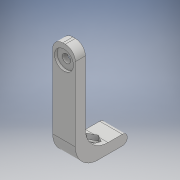
# Autodesk Inventor part: U2
Saved by Autodesk Inventor 2019 (Build 230136000, 136)
## iProperties
Part Number: U2
Material: Genérico
Document SubType Name: Modeling
Designer: beta3
Density: 1 g/cm^3
Appearance: Valor por defecto
Author: beta3
Autodesk Inventor part; units mm, degrees
ref_plane "YZ Plane" through (0, 0, 0) normal (1, 0, 0) x (0, 1, 0)
ref_plane "XZ Plane" through (0, 0, 0) normal (0, 1, 0) x (-1, 0, 0)
ref_plane "XY Plane" through (0, 0, 0) normal (0, 0, 1) x (1, 0, 0)
sketch "Boceto1" plane through (0, 0, 0) normal (0, 0, 1) x (1, 0, 0)
  line L0 (-13.5, 62) -> (13.5, 62)
  line L1 (13.5, 62) -> (13.5, 0)
  line L2 (13.5, 0) -> (-13.5, 0)
  line L3 (-13.5, 0) -> (-13.5, 62)
  line L4 (0, 0) -> (0, 62) construction
  line L5 (0, 40.815) -> (8.5, 35.9075)
  line L6 (8.5, 35.9075) -> (8.5, 26.0925)
  line L7 (8.5, 26.0925) -> (0, 21.185)
  line L8 (0, 21.185) -> (-8.5, 26.0925)
  line L9 (-8.5, 26.0925) -> (-8.5, 35.9075)
  line L10 (-8.5, 35.9075) -> (0, 40.815)
  line L11 (-8.5, 35.9075) -> (-13.5, 35.9075) construction
  line L12 (8.5, 35.9075) -> (13.5, 35.9075) construction
  point P0 (0, 31)
  dimension "d20" = 17
  dimension "d21" = 5
  dimension "d22" = 27
  dimension "d23" = 62
  constraints: 26 end point, 4 point on line, 3 midpoint, 2 parallel, 2 perpendicular, 1 horizontal, 1 symmetric about line, 1 vertical, 13 other
  measures "d20" distance between parallel lines of L6 L9
  measures "d21" distance of L9.end L11.end
  measures "d22" distance of L0.start L0.end
  measures "d23" distance of L2.end L0.start
extrude "Extrusión1" add sketch "Boceto1" along normal blind 6
sketch "Boceto2" plane through (0, 0, 0) normal (0, 0, -1) x (-1, 0, 0)
  line L0 (-8.5, 26.0925) -> (-8.5, 35.9075) projected
  line L1 (-8.5, 35.9075) -> (0, 40.815) projected
  line L2 (0, 40.815) -> (8.5, 35.9075) projected
  line L3 (8.5, 35.9075) -> (8.5, 26.0925) projected
  line L4 (8.5, 26.0925) -> (0, 21.185) projected
  line L5 (0, 21.185) -> (-8.5, 26.0925) projected
  line L6 (13.5, 62) -> (-13.5, 62) projected
  line L7 (-13.5, 62) -> (-13.5, 0) projected
  line L8 (-13.5, 0) -> (13.5, 0) projected
  line L9 (13.5, 0) -> (13.5, 62) projected
  point P0 (0, 0)
extrude "Extrusión2" add sketch "Boceto2" along normal blind 6 contours L0 L1 L2 L3 L4 L5 | L9 L8 L7 L6
sketch "Boceto3" plane through (0, 0, -6) normal (0, 0, -1) x (-1, 0, 0)
  line L0 (0, 0) -> (0, 62) construction
  line L1 (-13.5, 62) -> (13.5, 62) projected
  circle A0 centre (0, 31) radius 5.5
  dimension "d18" = 11
  constraints: 2 end point, 2 midpoint, 1 centre point
  measures "d18" diameter of A0
extrude "Extrusión3" cut sketch "Boceto3" against normal up to next
sketch "Boceto5" plane through (0, 0, 6) normal (0, 0, 1) x (1, 0, 0)
  line L0 (-13.5, 0) -> (-13.5, 62) projected
  line L1 (13.5, 62) -> (13.5, 0) projected
  line L2 (-13.5, 0) -> (13.5, 0)
  line L3 (13.5, 0) -> (13.5, 12)
  line L4 (13.5, 12) -> (-13.5, 12)
  line L5 (-13.5, 12) -> (-13.5, 0)
  line L6 (13.5, 62) -> (-13.5, 62) projected
  line L7 (-13.5, 62) -> (13.5, 62)
  line L8 (13.5, 62) -> (13.5, 50)
  line L9 (13.5, 50) -> (-13.5, 50)
  line L10 (-13.5, 50) -> (-13.5, 62)
  line L11 (-17.3027, 31) -> (12.0796, 31) construction
  line L12 (-8.5, 26.0925) -> (-8.5, 35.9075) projected
  point P0 (0, 0)
  point P1 (-8.5, 31)
  dimension "d24" = 12
  constraints: 18 end point, 4 parallel, 3 horizontal, 3 point on line, 2 perpendicular, 1 midpoint, 1 symmetric about line
  measures "d24" distance between parallel lines of L6 L9
extrude "Extrusión4" add sketch "Boceto5" along normal blind 115 contours L0 L4 L1 L2 | L0 L6 L1 L9
sketch "Boceto9" plane through (-13.5, 0, -6) normal (0, -1, 0) x (1, 0, 0)
  circle A0 centre (13.5, 110) radius 5
  line L0 (0, 127) -> (27, 127) projected
  line L1 (13.5, 110) -> (13.5, 115)
  line L2 (13.5, 115) -> (13.5, 127)
  line L3 (0, 127) -> (27, 127) projected
  point P0 (13.5, 6)
  dimension "d25" = 10
  dimension "d32" = 12
  constraints: 4 end point, 2 vertical, 1 midpoint, 1 vertical alignment, 2 other
  measures "d32" distance of L1.end L2.end
extrude "Extrusión8" cut sketch "Boceto9" against normal up to surface (12 mm away)
sketch "Boceto10" plane through (0, 0, -6) normal (0, 0, -1) x (-1, 0, 0)
  circle A0 centre (0, 31) radius 11
  circle A1 centre (0, 31) radius 5.5 projected
  point P0 (0, 0)
  dimension "d29" = 22
  constraints: 1 centre point, 1 coincident
  measures "d29" diameter of A0
extrude "Extrusión9" cut sketch "Boceto10" against normal blind 2.5
sketch "Boceto11" plane through (-13.5, 12, 6) normal (0, 1, 0) x (1, 0, 0)
  line L0 (21.5, -106) -> (5.5, -106) construction
  line L1 (5.5, -106) -> (5.5, -90) construction
  line L2 (5.5, -90) -> (21.5, -90) construction
  line L3 (21.5, -90) -> (21.5, -106) construction
  line L4 (5.5, -106) -> (21.5, -90) construction
  circle A0 centre (13.5, -98) radius 8 construction
  circle A1 centre (13.5, -98) radius 11.3137
  line L5 (27, 0) -> (27, -115) projected
  circle A2 centre (13.5, -98) radius 5 projected
  point P0 (13.5, 6)
  dimension "d45" = 16
  constraints: 10 end point, 3 coincident, 2 parallel, 2 perpendicular, 1 centre point, 1 horizontal, 1 midpoint, 1 tangent, 3 other
  measures "d45" distance of L2.end L0.start
extrude "Extrusión10" cut sketch "Boceto11" against normal blind 3 contours A1 | A2
sketch "Boceto12" plane through (-13.5, 0, -6) normal (0, -1, 0) x (1, 0, 0)
  circle A0 centre (13.5, 110) radius 11.3137 projected
  line L0 (0, 127) -> (0, 0) projected
  point P0 (13.5, 6)
  constraints: 1 coincident
extrude "Extrusión11" cut sketch "Boceto12" against normal blind 3
sketch "Boceto14" plane through (-13.5, 62, -6) normal (0, 1, 0) x (1, 0, 0)
  circle A0 centre (13.5, -110) radius 5 projected
  circle A1 centre (13.5, -110) radius 5
  point P0 (13.5, -6)
  dimension "d38" = 10
  constraints: 1 centre point, 1 coincident
  measures "d38" diameter of A1
extrude "Extrusión12" cut sketch "Boceto14" against normal up to next
sketch "Boceto15" plane through (-13.5, 50, 6) normal (0, -1, 0) x (1, 0, 0)
  circle A0 centre (13.5, 98) radius 5 projected
  circle A1 centre (13.5, 98) radius 12
  point P0 (13.5, -6)
  dimension "d41" = 24
  constraints: 1 centre point, 1 coincident
  measures "d41" diameter of A1
extrude "Extrusión13" cut sketch "Boceto15" against normal blind 8
fillet "Empalme4" radius 12 4 edges at (13.5, 56, 121) (-13.5, 56, 121) (13.5, 6, 121) (-13.5, 6, 121)
sketch "Boceto17" plane through (13.5, 12, 6) normal (1, 0, 0) x (0, 0, -1)
  line L0 (-103, 38) -> (-115, 38) projected
  line L1 (-103, 50) -> (12, 50) projected
  line L2 (-115, 38) -> (0, 38)
  line L3 (0, 38) -> (0, 50)
  line L4 (0, 50) -> (-115, 50)
  line L5 (-115, 50) -> (-115, 38)
  point P0 (6, -12)
  constraints: 8 end point, 2 parallel, 1 horizontal, 1 perpendicular
extrude "Extrusión14" cut sketch "Boceto17" against normal up to next
fillet "Empalme7" radius 6 2 edges at (0, 62, -6) (0, 62, 6)
fillet "Empalme8" radius 27 1 edges at (0, 12, 6)
fillet "Empalme9" radius 27 1 edges at (0, 0, -6)
